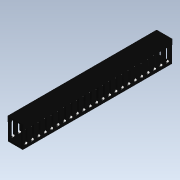
# Autodesk Inventor part: Kabelkanal_25x50_400
Saved by Autodesk Inventor 2022.2 (Build 262287000, 287)
## iProperties
Created: 2021-12-01
Part Number: Kabelkanal_25x50_400
Material: Generic
Document SubType Name: Modeling
Designer: Fabijan_Sven
Density: 1 g/cm^3
Appearance: Default
Author: Fabijan_Sven
Autodesk Inventor part; units mm, degrees
ref_plane "YZ Plane" through (0, 0, 0) normal (1, 0, 0) x (0, 1, 0)
ref_plane "XZ Plane" through (0, 0, 0) normal (0, 1, 0) x (-1, 0, 0)
ref_plane "XY Plane" through (0, 0, 0) normal (0, 0, 1) x (1, 0, 0)
sketch "Sketch1" plane through (0, 0, 0) normal (0, 0, 1) x (1, 0, 0)
  line L0 (0, 0) -> (25, 0)
  line L1 (25, 0) -> (25, 28.7883)
  line L2 (0, 28.7883) -> (2, 33.5)
  line L3 (2, 33.5) -> (0, 33.5)
  line L4 (0, 35.5) -> (4.5, 35.5)
  line L5 (4.5, 35.5) -> (4.5, 32.3221)
  line L6 (4.5, 32.3221) -> (3, 28.7883)
  line L7 (3, 28.7883) -> (3, 3)
  line L8 (3, 3) -> (22, 3)
  line L9 (22, 3) -> (22, 28.7883)
  line L10 (22, 28.7883) -> (20.5, 32.3221)
  line L11 (20.5, 32.3221) -> (20.5, 35.5)
  line L12 (20.5, 35.5) -> (25, 35.5)
  line L13 (0, 35.5) -> (0, 33.5)
  line L14 (0, 28.7883) -> (0, 0)
  line L15 (25, 33.5) -> (25, 35.5)
  line L16 (-11.0413, 28.7883) -> (46.5378, 28.7883) construction
  line L17 (25, 28.7883) -> (23, 33.5)
  line L18 (23, 33.5) -> (25, 33.5)
  dimension "d2" = 2
  dimension "d3" = 35.5
  dimension "d5" = 67
  dimension "d6" = 67
  dimension "d7" = 4.5
  dimension "d8" = 4.5
  dimension "d9" = 25
  dimension "d10" = 3
  dimension "d11" = 3
  dimension "d12" = 3
  dimension "d13" = 2
  dimension "d33" = 2
  constraints: 38 end point, 9 point on line, 7 parallel, 7 perpendicular, 4 horizontal
  measures "d2" distance from line of L14 L2.end
  measures "d3" distance between parallel lines of L0 L12
  measures "d5" angle of L6 L16
  measures "d6" angle of L16 L10
  measures "d7" distance between parallel lines of L13 L5
  measures "d8" distance between parallel lines of L11 L15
  measures "d9" distance between parallel lines of L14 L1
  measures "d10" distance between parallel lines of L0 L8
  measures "d11" distance between parallel lines of L14 L7
  measures "d12" distance between parallel lines of L1 L9
  measures "d13" distance of L17.end L15.start
  measures "d33" distance between parallel lines of L12 L18
extrude "Extrusion1" add sketch "Sketch1" along normal blind 255
sketch "Sketch2" plane through (0, 0, 0) normal (-1, 0, 0) x (0, 0, 1)
  line L0 (7, 35) -> (8, 35)
  line L1 (10, 33) -> (10, 7)
  line L2 (8, 5) -> (7, 5)
  line L3 (5, 7) -> (5, 33)
  line L4 (0, 0) -> (255, 0) projected
  line L5 (0, 28.7883) -> (0, 0) projected
  arc A0 (7, 35) -> (5, 33) centre (7, 33) ccw
  arc A1 (10, 33) -> (8, 35) centre (8, 33) ccw
  arc A2 (5, 7) -> (7, 5) centre (7, 7) ccw
  arc A3 (8, 5) -> (10, 7) centre (8, 7) ccw
  point P0 (5, 35)
  point P1 (10, 5)
  point P2 (10, 35)
  point P3 (5, 5)
  dimension "d16" = 5
  dimension "d17" = 30
  dimension "d18" = 5
  dimension "d19" = 5
  dimension "d30" = 2
  constraints: 8 end point, 8 point on circle, 8 point on line, 8 tangent, 4 centre point, 3 equal radius, 2 parallel, 1 horizontal, 1 perpendicular
  measures "d16" distance of point (5, 35) point (10, 35)
  measures "d17" distance between parallel lines of L2 L0
  measures "d18" distance between parallel lines of L4 L2
  measures "d19" distance between parallel lines of L5 L3
  measures "d30" radius of A0
extrude "Extrusion2" cut sketch "Sketch2" against normal blind 500
pattern_linear "Rectangular Pattern1" count 60 spacing 11 along (0, 0, 1) of "Extrusion2"
sketch "Sketch3" plane through (0, 0, 0) normal (0, 0, -1) x (-1, 0, 0)
  line L0 (-25, 28.7883) -> (-23, 33.5) projected
  line L1 (-23, 33.5) -> (-25, 28.7883)
  line L2 (-25, 28.7883) -> (-26, 28.7883)
  line L3 (-26, 28.7883) -> (-26, 37.5)
  line L4 (-26, 37.5) -> (1, 37.5)
  line L5 (1, 37.5) -> (1, 28.7883)
  line L6 (1, 28.7883) -> (0, 28.7883)
  line L7 (0, 33.5) -> (-2, 33.5) projected
  line L8 (0, 28.7883) -> (-2, 33.5)
  line L9 (-2, 33.5) -> (0, 33.5)
  line L10 (-4.5, 35.5) -> (0, 35.5) projected
  line L11 (0, 33.5) -> (0, 35.5)
  line L12 (0, 35.5) -> (-4.5, 35.5)
  line L13 (-25, 35.5) -> (-20.5, 35.5) projected
  line L14 (-4.5, 35.5) -> (-25, 35.5)
  line L15 (-23, 33.5) -> (-25, 33.5) projected
  line L16 (-25, 35.5) -> (-25, 33.5)
  line L17 (-25, 33.5) -> (-23, 33.5)
  line L18 (-23, 33.5) -> (-25, 28.7883)
  line L19 (0, 0) -> (-25, 0) projected
  line L20 (-4.5, 35.5) -> (0, 35.5) projected
  point P0 (-2.25, 35.5)
  dimension "d26" = 1
  dimension "d27" = 1
  dimension "d32" = 2
  constraints: 28 end point, 7 perpendicular, 4 collinear, 1 horizontal, 1 midpoint, 1 point on line
  measures "d26" distance between parallel lines of L16 L3
  measures "d27" distance between parallel lines of L11 L5
  measures "d32" distance from line of point (-2.25, 35.5) L4
extrude "Extrusion3" add sketch "Sketch3" against normal up to surface (255 mm away)
body "Solid1"
